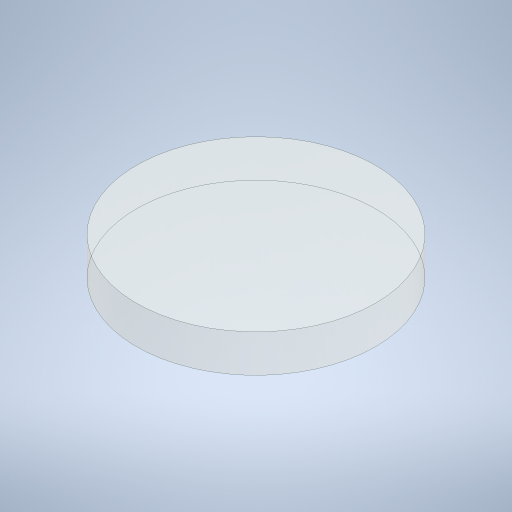
# Autodesk Inventor part: Fenster Kamera
Saved by Autodesk Inventor 2024 (Build 280153000, 153)
## iProperties
Created: 2024-03-04
Part Number: Fenster Kamera
Material: Glas
Document SubType Name: Modeling
Designer: Andreas Weber
Mass: 0.828467 g
Surface Area: 3.73048 cm^2
Volume: 0.380031 cm^3
Density: 2.18 g/cm^3
Appearance: Klar
Author: Andreas Weber
Autodesk Inventor part; units mm, degrees
ref_plane "YZ Plane" through (0, 0, 0) normal (1, 0, 0) x (0, 1, 0)
ref_plane "XZ Plane" through (0, 0, 0) normal (0, 1, 0) x (-1, 0, 0)
ref_plane "XY Plane" through (0, 0, 0) normal (0, 0, 1) x (1, 0, 0)
sketch "Skizze2" plane through (0, 0, 0) normal (0, 0, 1) x (1, 0, 0)
  circle A0 centre (0, 0) radius 6.35
  dimension "d3" = 12.7
  constraints: 1 centre point, 1 coincident
  measures "d3" diameter of A0
extrude "Extrusion2" add sketch "Skizze2" along normal blind 2
